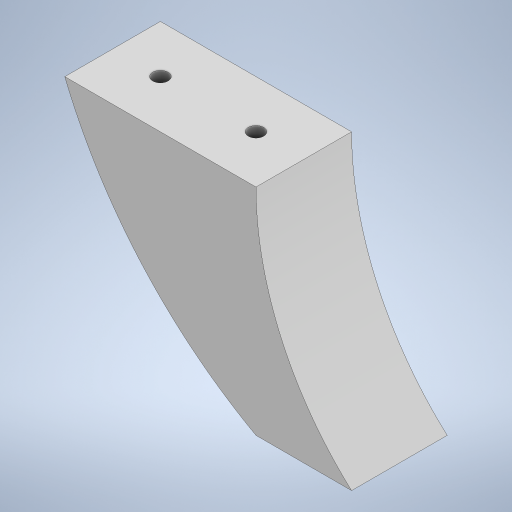
# Autodesk Inventor part: Feet
Saved by Autodesk Inventor 2023.1 (Build 271208000, 208)
## iProperties
Created: 2022-11-07
Part Number: Feet
Material: Generic
Document SubType Name: Modeling
Designer: nicol
Density: 1 g/cm^3
Appearance: Default
Author: nicol
Autodesk Inventor part; units mm, degrees
ref_plane "YZ Plane" through (0, 0, 0) normal (1, 0, 0) x (0, 1, 0)
ref_plane "XZ Plane" through (0, 0, 0) normal (0, 1, 0) x (-1, 0, 0)
ref_plane "XY Plane" through (0, 0, 0) normal (0, 0, 1) x (1, 0, 0)
sketch "Sketch1" plane through (0, 0, 0) normal (0, 0, 1) x (1, 0, 0)
  line L0 (0, 0) -> (20, 0)
  line L1 (-40, 45) -> (0, 45)
  arc A0 (-40, 45) -> (0, 0) centre (43.3923, 78.8487) ccw
  arc A1 (0, 45) -> (20, 0) centre (60.625, 45) ccw
  line L2 (0, 45) -> (0, 29.5126) construction
  line L3 (-40, 45) -> (-40, 23.133) construction
  dimension "d0" = 45
  dimension "d1" = 20
  dimension "d2" = 40
  dimension "d3" = 90
  constraints: 8 end point, 4 point on circle, 2 centre point, 2 horizontal, 2 vertical, 1 tangent, 1 vertical alignment
  measures "d0" distance between parallel lines of L0 L1
  measures "d1" distance of L0.start L0.end
  measures "d2" distance of L1.start L1.end
  measures "d3" radius of A0
extrude "Extrusion1" add sketch "Sketch1" along normal blind 20
ref_plane "Work Plane1" through (-40, 40, 0) normal (0, 1, 0) x (1, 0, 0)
sketch "Sketch2" plane through (-40, 45, 0) normal (0, 1, 0) x (1, 0, 0)
  line L0 (40, 0) -> (40, -20) projected
  line L1 (0, 0) -> (0, -20) projected
  circle A0 centre (10, -10) radius 3.25
  circle A1 centre (30, -10) radius 3.25
  point P0 (0, -10)
  dimension "d7" = 10
  dimension "d8" = 10
  dimension "d9" = 6.5
  dimension "d10" = 6.5
  constraints: 2 centre point, 2 coincident, 2 horizontal alignment, 1 midpoint
  measures "d7" distance from line of L0 point (30, -10)
  measures "d8" distance from line of L1 point (10, -10)
  measures "d9" diameter of A0
  measures "d10" diameter of A1
hole "Hole1" at (-30, 45, 10) at (-10, 45, 10) direction (0, -1, 0) diameter 3.2 end through all
extrude "Extrusion2" cut sketch "Sketch2" against normal blind 58.25 from surface at -5
body "Solid1"
